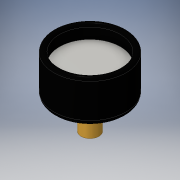
# Autodesk Inventor part: Z1000
Saved by Autodesk Inventor 2016 SP2 (Build 200236200, 236)
## iProperties
Created: 2017-03-30
Part Number: Z1000
Material: Aluminum
Document SubType Name: Modeling
Designer: smiku
Mass: 69.038 g
Surface Area: 70.368 cm^2
Volume: 25.5696 cm^3
Density: 2.7 g/cm^3
Appearance: Anodized - Black
Author: smiku
Autodesk Inventor part; units mm, degrees
ref_plane "YZ Plane" through (0, 0, 0) normal (1, 0, 0) x (0, 1, 0)
ref_plane "XZ Plane" through (0, 0, 0) normal (0, 1, 0) x (-1, 0, 0)
ref_plane "XY Plane" through (0, 0, 0) normal (0, 0, 1) x (1, 0, 0)
sketch "Sketch1" plane through (0, 0, 0) normal (0, 1, 0) x (-1, 0, 0)
  circle A0 centre (0, 0) radius 20.447
  dimension "d0" = 40.894
  constraints: 1 centre point, 1 coincident
  measures "d0" diameter of A0
extrude "Extrusion1" add sketch "Sketch1" along normal blind 24.003
sketch "Sketch2" plane through (0, 24.003, 0) normal (0, 1, 0) x (1, 0, 0)
  circle A0 centre (0, 0) radius 17.272
  circle A1 centre (0, 0) radius 20.447 projected
  dimension "d6" = 3.175
  constraints: 1 centre point, 1 coincident
  measures "d6" radial gap between concentric circles of A1 A0
extrude "Extrusion2" cut sketch "Sketch2" against normal blind 7.62 contours A0
fillet "Fillet1" radius 3.175 1 edges at (20.447, 0, 0)
fillet "Fillet2" radius 1.5875 2 edges at (-17.272, 24.003, 0) (20.447, 24.003, 0)
sketch "Sketch3" plane through (0, 0, 0) normal (0, -1, 0) x (1, 0, 0)
  line L0 (-5.461, -5.461) -> (5.461, -5.461)
  line L1 (5.461, -5.461) -> (5.461, 5.461)
  line L2 (5.461, 5.461) -> (-5.461, 5.461)
  line L3 (-5.461, 5.461) -> (-5.461, -5.461)
  line L4 (-5.461, -5.461) -> (5.461, 5.461) construction
  line L5 (5.461, -5.461) -> (-5.461, 5.461) construction
  point P0 (0, 0)
  dimension "d9" = 10.922
  dimension "d10" = 10.922
  constraints: 12 end point, 2 midpoint, 2 parallel, 1 horizontal, 1 perpendicular
  measures "d9" distance of L2.end L1.end
  measures "d10" distance of L1.end L0.end
extrude "Extrusion3" add sketch "Sketch3" along normal blind 6.35 separate body
sketch "Sketch4" plane through (0, -6.35, 0) normal (0, -1, 0) x (1, 0, 0)
  circle A0 centre (0, 0) radius 5.08
  dimension "d13" = 10.16
  constraints: 1 centre point, 1 coincident
  measures "d13" diameter of A0
extrude "Extrusion4" add sketch "Sketch4" along normal blind 10.16 bodies 2
body "Solid1"
body "Solid2"
